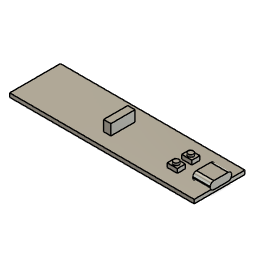
bottom_cover (1) v7 (Autodesk Fusion 360 archive; units mm, degrees)
design "Pico LiPo 2 XL W"
Autodesk Fusion 360 part; units mm, degrees
note: some values were not read from the file. Chosen so that the rebuilt part matches the saved one: which bodies a step acts on.
sketch "Base" plane through (0, 0, 0) normal (0, 1, 0) x (1, 0, 0) in component "Pico LiPo 2 XL W"
  line L0 (38.2, -10.5) -> (-38.2, -10.5)
  line L1 (-38.2, -10.5) -> (-38.2, 10.5)
  line L2 (-38.2, 10.5) -> (38.2, 10.5)
  line L3 (38.2, 10.5) -> (38.2, -10.5)
  line L4 (38.2, -10.5) -> (-38.2, 10.5) construction
  line L5 (-38.2, -10.5) -> (38.2, 10.5) construction
  line L6 (38.2, 0) -> (-38.2, 0)
  line L7 (31.6, 4.45) -> (38.8, 4.45)
  line L8 (38.8, 4.45) -> (38.8, -4.45)
  line L9 (38.8, -4.45) -> (31.6, -4.45)
  line L10 (31.6, -4.45) -> (31.6, 4.45)
  line L11 (21.2, 4.65) -> (25.4, 4.65)
  line L12 (25.4, 4.65) -> (25.4, 1.35)
  line L13 (25.4, 1.35) -> (21.2, 1.35)
  line L14 (21.2, 1.35) -> (21.2, 4.65)
  line L15 (25.4, -4.65) -> (25.4, -1.35)
  line L16 (21.2, -4.65) -> (25.4, -4.65)
  line L17 (25.4, -1.35) -> (21.2, -1.35)
  line L18 (21.2, -1.35) -> (21.2, -4.65)
  line L19 (-4.8, 5) -> (-1.8, 5)
  line L20 (-1.8, 5) -> (-1.8, -5)
  line L21 (-1.8, -5) -> (-4.8, -5)
  line L22 (-4.8, -5) -> (-4.8, 5)
  dimension "d1" = 76.4
  dimension "d2" = 21
  dimension "d3" = 7.2
  dimension "d4" = 8.9
  dimension "d5" = 0.6
  dimension "d6" = 8.9
  dimension "d7" = 3.3
  dimension "d8" = 4.2
  dimension "d9" = 9.3
  dimension "d10" = 17
  dimension "d11" = 40
  dimension "d12" = 3
  dimension "d13" = 10
  dimension "d14" = 10
  constraint horizontal L0
  constraint perpendicular L0 L1
  constraint parallel L0 L2
  constraint parallel L1 L3
  constraint coincident L4 origin
  constraint coincident L5 origin
  constraint midpoint L3 L6.start
  constraint midpoint L1 L6.end
  constraint horizontal L7
  constraint vertical L8
  constraint horizontal L9
  constraint vertical L10
  constraint horizontal L11
  constraint vertical L12
  constraint horizontal L13
  constraint vertical L14
  constraint symmetric L6 L11.start L16.start
  constraint symmetric L6 L11.end L15.start
  constraint symmetric L6 L12.end L15.end
  constraint symmetric L6 L13.end L17.end
  constraint horizontal L19
  constraint vertical L20
  constraint horizontal L21
  constraint vertical L22
  measures "d1" distance of L1.end L2.end
  measures "d2" distance of L0.end L1.end
  measures "d3" distance of L7.start L7.end
  measures "d4" distance of L7.start L9.end
  measures "d5" distance of L3 L8
  measures "d7" distance of L11 L13
  measures "d8" distance of L12 L14
  measures "d10" distance of L3 L14
  measures "d11" distance of L3 L20
  measures "d12" distance of L20 L22
  measures "d13" distance of L19 L21
extrude "Extrude1" add sketch "Base" along normal blind 1.6 contours L0 L1 L3 L6 L9 L10 L20 L21 L22 | L3 L6 L9 L10 | L1 L2 L3 L6 L7 L10 L19 L20 L22 | L3 L6 L7 L10 | L6 L19 L20 L22 | L6 L20 L21 L22 | L11 L12 L13 L14 | L15 L16 L17 L18 makes body 1 in component "Pico LiPo 2 XL W"
extrude "Extrude2" add sketch "Base" along normal blind 3.25 from surface at 1.6 contours L3 L6 L9 L10 | L3 L7 L8 L9 | L3 L6 L7 L10 bodies 1 in component "Pico LiPo 2 XL W"
extrude "Extrude3" add sketch "Base" along normal blind 1.7 from surface at 1.6 contours L11 L12 L13 L14 | L15 L16 L17 L18 bodies 1 in component "Pico LiPo 2 XL W"
extrude "Extrude4" add sketch "Base" along normal blind 4.4 from surface at 1.6 contours L6 L19 L20 L22 | L6 L20 L21 L22 bodies 1 in component "Pico LiPo 2 XL W"
ref_plane "WorkPlane1" through (0, 1.6, 0) normal (0, 1, 0) x (0, 0, 1) in component "Pico LiPo 2 XL W"
split "Split1" by plane through (0, 1.6, 0) normal (0, 1, 0) bodies 1 makes body 2 at (24, 3.3, 3.55) makes body 3 at (34, 4.85, -1.4833) makes body 4 at (22.6, 3.3, -3.55) makes body 5 at (-4.8, 4.5333, -1.6667) in component "Pico LiPo 2 XL W"
fillet "Fillet1" radius 1.5 2 edges at (35.2, 4.85, -4.45) (35.2, 1.6, -4.45) on bodies 3 in component "Pico LiPo 2 XL W"
fillet "Fillet2" radius 1.5 2 edges at (35.2, 1.6, 4.45) (35.2, 4.85, 4.45) on bodies 3 in component "Pico LiPo 2 XL W"
combine "Combine1" operation add target body 5 tool bodies 2 4 3 1 in component "Pico LiPo 2 XL W"
sketch "buttons" plane through (0, 3.3, 0) normal (0, 1, 0) x (-1, 0, 0) in component "Pico LiPo 2 XL W"
  line L0 (-21.2, -1.35) -> (-25.4, -1.35)
  line L1 (-25.4, -1.35) -> (-25.4, -4.65)
  line L2 (-25.4, -4.65) -> (-21.2, -4.65)
  line L3 (-21.2, -4.65) -> (-21.2, -1.35)
  line L4 (-25.4, -4.65) -> (-21.2, -4.65)
  line L5 (-25.4, -1.35) -> (-25.4, -4.65)
  line L6 (-21.2, -1.35) -> (-25.4, -1.35)
  line L7 (-21.2, -4.65) -> (-21.2, -1.35)
  line L8 (-25.4, 4.65) -> (-25.4, 1.35)
  line L9 (-25.4, 1.35) -> (-21.2, 1.35)
  line L10 (-21.2, 1.35) -> (-21.2, 4.65)
  line L11 (-21.2, 4.65) -> (-25.4, 4.65)
  line L12 (-21.2, -3) -> (-25.4, -3)
  line L13 (-23.3, -4.65) -> (-23.3, -1.35)
  line L14 (-23.3, 1.35) -> (-23.3, 4.65)
  line L15 (-21.2, 3) -> (-25.4, 3)
  circle A0 centre (-23.3, -3) radius 1.125
  circle A1 centre (-23.3, 3) radius 1.125
  dimension "d31" = 2.25
  dimension "d32" = 2.25
  constraint midpoint L7 L12.start
  constraint midpoint L5 L12.end
  constraint midpoint L4 L13.start
  constraint midpoint L6 L13.end
  constraint midpoint L9 L14.start
  constraint midpoint L11 L14.end
  constraint midpoint L10 L15.start
  constraint midpoint L8 L15.end
  constraint midpoint L13 A0.centre
  constraint midpoint L15 A1.centre
  measures "d31" diameter of A0
  measures "d32" diameter of A1
extrude "Extrude5" add sketch "buttons" along normal blind 0.9 contours L12 L13 A0 | L12 L13 A0 | L12 L13 A0 | L12 L13 A0 | L14 L15 A1 | L14 L15 A1 | L14 L15 A1 | L14 L15 A1 bodies 5 in component "Pico LiPo 2 XL W"
component "Pico LiPo 2 XL W" placed x (1, 0, 0) y (0, 1, 0) z (0, 0, 1) at (0, 0, 0)
equation "d14 = d13"
equation "d21 = 3.3 mm - 1.6 mm"
equation "d24 = 6 mm - 1.6 mm"
named bodies: "PCB"
